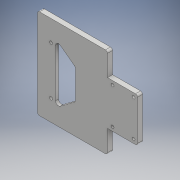
# Autodesk Inventor part: drzaksolaru
Saved by Autodesk Inventor 2017 (Build 210142000, 142)
## iProperties
Created: 2019-02-02
Part Number: drzaksolaru
Material: Generic
Document SubType Name: Modeling
Designer: Denis Kurka
Density: 1 g/cm^3
Appearance: Default
Author: Denis Kurka
Autodesk Inventor part; units mm, degrees
ref_plane "YZ Plane" through (0, 0, 0) normal (1, 0, 0) x (0, 1, 0)
ref_plane "XZ Plane" through (0, 0, 0) normal (0, 1, 0) x (-1, 0, 0)
ref_plane "XY Plane" through (0, 0, 0) normal (0, 0, 1) x (1, 0, 0)
sketch "Sketch1" plane through (0, 0, 0) normal (0, 1, 0) x (-1, 0, 0)
  line L0 (0, 0) -> (70, 0)
  line L1 (70, 0) -> (70, -90)
  line L2 (70, -90) -> (0, -90)
  line L3 (0, -90) -> (0, 0)
  line L4 (0, -67) -> (-30, -67)
  line L5 (-30, -67) -> (-30, -23)
  line L6 (-30, -23) -> (0, -23)
  line L7 (0, -23) -> (0, -67)
  dimension "d0" = 70
  dimension "d1" = 90
  dimension "d2" = 44
  dimension "d3" = 30
  dimension "d4" = 23
  dimension "d5" = 23
  constraints: 16 end point, 4 parallel, 2 horizontal, 2 perpendicular, 1 point on line
  measures "d0" distance of L1.end L2.end
  measures "d1" distance of L0.end L1.end
  measures "d2" distance of L4.end L5.end
  measures "d3" distance of L4.start L4.end
  measures "d4" distance between parallel lines of L0 L6
  measures "d5" distance between parallel lines of L2 L4
extrude "Extrusion1" add sketch "Sketch1" along normal blind 5
sketch "Sketch2" plane through (0, 5, 0) normal (0, 1, 0) x (1, 0, 0)
  line L0 (-67, 3) -> (-3, 3)
  line L1 (-3, 3) -> (-3, 87)
  line L2 (-3, 87) -> (-67, 87)
  line L3 (-67, 87) -> (-67, 3)
  line L4 (-70, 0) -> (0, 0) projected
  line L5 (-70, 90) -> (-70, 0) projected
  line L6 (0, 90) -> (-70, 90) projected
  line L7 (0, 0) -> (0, 23) projected
  dimension "d8" = 3
  dimension "d10" = 3
  dimension "d12" = 3
  dimension "d13" = 3
  constraints: 8 end point, 2 parallel, 1 horizontal, 1 perpendicular
  measures "d8" distance between parallel lines of L4 L0
  measures "d10" distance between parallel lines of L5 L3
  measures "d12" distance between parallel lines of L6 L2
  measures "d13" distance between parallel lines of L7 L1
extrude "Extrusion2" cut sketch "Sketch2" against normal blind 2
sketch "Sketch3" plane through (0, 3, 0) normal (0, 1, 0) x (1, 0, 0)
  line L0 (-52, 15) -> (-52, 75)
  line L1 (-52, 15) -> (-32, 30)
  line L2 (-32, 30) -> (-32, 60)
  line L3 (-32, 60) -> (-52, 75)
  line L4 (-67, 3) -> (-67, 87) projected
  line L5 (-3, 3) -> (-67, 3) projected
  line L6 (-67, 87) -> (-3, 87) projected
  circle A0 centre (-56.4262, 20.9016) radius 1.5
  circle A1 centre (-56.4262, 69.0984) radius 1.5
  point P0 (0, 0)
  dimension "d16" = 60
  dimension "d17" = 30
  dimension "d18" = 15
  dimension "d19" = 20
  dimension "d20" = 27
  dimension "d21" = 27
  dimension "d22" = 12
  dimension "d23" = 12
  dimension "d24" = 3
  dimension "d25" = 3
  constraints: 8 end point, 2 centre point, 1 vertical
  measures "d16" distance of L0.start L0.end
  measures "d17" distance of L1.end L2.end
  measures "d18" distance between parallel lines of L0 L4
  measures "d19" distance between parallel lines of L2 L0
  measures "d20" distance from line of L5 L1.end
  measures "d21" distance from line of L6 L2.end
  measures "d22" distance from line of L5 L0.start
  measures "d23" distance from line of L6 L0.end
  measures "d24" diameter of A0
  measures "d25" diameter of A1
extrude "Extrusion3" cut sketch "Sketch3" against normal blind 10
fillet "Fillet1" radius 3 4 edges at (-52, 1.5, -15) (-32, 1.5, -30) (-32, 1.5, -60) (-52, 1.5, -75)
fillet "Fillet2" radius 2 6 edges at (0, 2.5, 0) (0, 2.5, -90) (-70, 2.5, -90) (-70, 2.5, 0) (30, 2.5, -23) (30, 2.5, -67)
sketch "Sketch4" plane through (0, 5, 0) normal (0, 1, 0) x (1, 0, 0)
  circle A0 centre (26.1, 26.9) radius 1.5
  line L0 (30, 25) -> (30, 65) projected
  line L1 (0, 23) -> (28, 23) projected
  circle A1 centre (26.1, 63.1) radius 1.5
  line L2 (28, 67) -> (0, 67) projected
  circle A2 centre (5.1, 26.9) radius 1.5
  circle A3 centre (5.1, 63.1) radius 1.5
  point P0 (0, 0)
  dimension "d30" = 3
  dimension "d31" = 3.9
  dimension "d32" = 3.9
  dimension "d33" = 3
  dimension "d34" = 3.9
  dimension "d35" = 3.9
  dimension "d36" = 3
  dimension "d37" = 21
  dimension "d38" = 3
  dimension "d39" = 21
  dimension "d40" = 3.9
  dimension "d41" = 3.9
  constraints: 4 centre point
  measures "d30" diameter of A0
  measures "d31" distance from line of L0 A0.centre
  measures "d32" distance from line of A0.centre L1
  measures "d33" diameter of A1
  measures "d34" distance from line of L2 A1.centre
  measures "d35" distance from line of L0 A1.centre
  measures "d36" diameter of A2
  measures "d37" distance of A0.centre A2.centre
  measures "d38" diameter of A3
  measures "d39" distance of A1.centre A3.centre
  measures "d40" distance from line of L2 A3.centre
  measures "d41" distance from line of L1 A2.centre
extrude "Extrusion4" cut sketch "Sketch4" against normal blind 10
equation "\"d4\" = d5"
equation "\"d20\" = d21"
equation "\"d22\" = d23"
body "Solid1"
